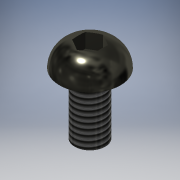
# Autodesk Inventor part: SB　M4 8mm なべネジ
Saved by Autodesk Inventor 2017.3 (Build 213256000, 256)
## iProperties
Created: 2014-02-17
Part Number: SB　M4 8mm なべネジ
Material: Stainless Steel, 440C
Document SubType Name: Modeling
Designer: shiota
Mass: 1.51458 g
Surface Area: 2.60244 cm^2
Volume: 0.195429 cm^3
Density: 7.75 g/cm^3
Appearance: ガンメタル
Author: shiota
Autodesk Inventor part; units mm, degrees
ref_plane "YZ Plane" through (0, 0, 0) normal (1, 0, 0) x (0, 1, 0)
ref_plane "XZ Plane" through (0, 0, 0) normal (0, 1, 0) x (-1, 0, 0)
ref_plane "XY Plane" through (0, 0, 0) normal (0, 0, 1) x (1, 0, 0)
sketch "スケッチ1" plane through (0, 0, 0) normal (0, 0, 1) x (1, 0, 0)
  circle A0 centre (0, 0) radius 2
  dimension "d0" = 4
  constraints: 1 centre point, 1 coincident
  measures "d0" diameter of A0
extrude "押し出し1" add sketch "スケッチ1" along normal blind 8
sketch "スケッチ2" plane through (0, 0, 8) normal (0, 0, 1) x (1, 0, 0)
  circle A0 centre (0, 0) radius 2 projected
  circle A1 centre (0, 0) radius 4
  dimension "d3" = 8
  constraints: 1 centre point, 1 coincident
  measures "d3" diameter of A1
extrude "押し出し2" add sketch "スケッチ2" along normal blind 3 contours A0 | A1
fillet "フィレット1" radius 3 1 edges at (-4, 0, 11)
thread "ねじ1" size "M4x0.7" class "6g" standard "ANSI Metric M Profile" full length
sketch "スケッチ3" plane through (0, 0, 11) normal (0, 0, 1) x (1, 0, 0)
  line L0 (-1.5, 0.866) -> (0, 1.7321)
  line L1 (0, 1.7321) -> (1.5, 0.866)
  line L2 (1.5, 0.866) -> (1.5, -0.866)
  line L3 (1.5, -0.866) -> (0, -1.7321)
  line L4 (0, -1.7321) -> (-1.5, -0.866)
  line L5 (-1.5, -0.866) -> (-1.5, 0.866)
  point P0 (0, 0)
  point P1 (0, 0)
  point P2 (-1.5, 0)
  dimension "d9" = 3
  constraints: 12 end point, 1 coincident, 1 midpoint, 1 vertical, 13 other
  measures "d9" distance between parallel lines of L2 L5
extrude "押し出し3" cut sketch "スケッチ3" against normal blind 2
